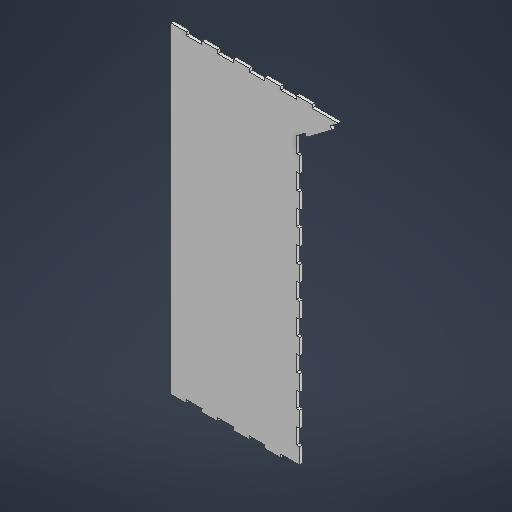
# Autodesk Inventor part: side
Saved by Autodesk Inventor 2026 (Build 300175050, 175E)
## iProperties
Created: 2025-08-08
Part Number: side
Material: Genérico
Document SubType Name: Modeling
Designer: EspacoMaker
Density: 1 g/cm^3
Appearance: Padrão
Author: EspacoMaker
Autodesk Inventor part; units mm, degrees
ref_plane "YZ Plane" through (0, 0, 0) normal (1, 0, 0) x (0, 1, 0)
ref_plane "XZ Plane" through (0, 0, 0) normal (0, 1, 0) x (-1, 0, 0)
ref_plane "XY Plane" through (0, 0, 0) normal (0, 0, 1) x (1, 0, 0)
sketch "Esboço1" plane through (0, 0, 0) normal (0, 0, 1) x (1, 0, 0)
  line L0 (60, -135) -> (-60, -135)
  line L1 (-60, -135) -> (-60, 135)
  line L2 (-60, 135) -> (60, 135)
  line L3 (60, 135) -> (60, -135)
  line L4 (60, -135) -> (-60, 135) construction
  line L5 (-60, -135) -> (60, 135) construction
  line L6 (-60, 135) -> (60, 135)
  line L7 (60, 135) -> (60, 165)
  line L8 (60, 165) -> (-60, 165)
  line L9 (-60, 165) -> (-60, 135)
  line L10 (60, 165) -> (100, 165)
  line L11 (100, 165) -> (60, 135)
  point P0 (0, 0)
  dimension "d0" = 120
  dimension "d1" = 270
  dimension "d2" = 120
  dimension "d3" = 30
  dimension "d4" = 40
  constraints: 24 end point, 4 parallel, 3 horizontal, 2 midpoint, 2 perpendicular
  measures "d0" distance of L1.end L2.end
  measures "d1" distance of L0.end L1.end
  measures "d2" distance of L8.end L7.end
  measures "d3" distance of L7.end L6.end
  measures "d4" distance of L7.end L10.end
extrude "Extrusão1" add sketch "Esboço1" along normal blind 3
sketch "Esboço2" plane through (60, -135, 0) normal (1, 0, 0) x (0, 0, -1)
  line L0 (-3, 0) -> (0, 0)
  line L1 (0, 0) -> (0, 15)
  line L2 (0, 15) -> (-3, 15)
  line L3 (-3, 15) -> (-3, 0)
  line L4 (-3, 30) -> (0, 30)
  line L5 (0, 30) -> (0, 45)
  line L6 (0, 45) -> (-3, 45)
  line L7 (-3, 45) -> (-3, 30)
  line L8 (-3, 60) -> (0, 60)
  line L9 (0, 60) -> (0, 75)
  line L10 (0, 75) -> (-3, 75)
  line L11 (-3, 75) -> (-3, 60)
  line L12 (-3, 90) -> (0, 90)
  line L13 (0, 90) -> (0, 105)
  line L14 (0, 105) -> (-3, 105)
  line L15 (-3, 105) -> (-3, 90)
  line L16 (-3, 120) -> (0, 120)
  line L17 (0, 120) -> (0, 135)
  line L18 (0, 135) -> (-3, 135)
  line L19 (-3, 135) -> (-3, 120)
  line L20 (-3, 150) -> (0, 150)
  line L21 (0, 150) -> (0, 165)
  line L22 (0, 165) -> (-3, 165)
  line L23 (-3, 165) -> (-3, 150)
  line L24 (-3, 180) -> (0, 180)
  line L25 (0, 180) -> (0, 195)
  line L26 (0, 195) -> (-3, 195)
  line L27 (-3, 195) -> (-3, 180)
  line L28 (-3, 210) -> (0, 210)
  line L29 (0, 210) -> (0, 225)
  line L30 (0, 225) -> (-3, 225)
  line L31 (-3, 225) -> (-3, 210)
  line L32 (-3, 240) -> (0, 240)
  line L33 (0, 240) -> (0, 255)
  line L34 (0, 255) -> (-3, 255)
  line L35 (-3, 255) -> (-3, 240)
  dimension "d7" = 3
  dimension "d8" = 15
  dimension "d11" = 30
  constraints: 72 end point, 2 parallel, 1 collinear, 1 horizontal, 1 perpendicular, 1 vertical, 63 other
  measures "d7" distance of L2.end L1.end
  measures "d8" distance of L1.end L0.end
  measures "d11" distance of L1.end L5.end
sketch "Esboço3" plane through (-60, -135, 0) normal (0, -1, 0) x (1, 0, 0)
  line L0 (160, 3) -> (0, 3) projected
  line L1 (0, 0) -> (15, 0)
  line L2 (15, 0) -> (15, 3)
  line L3 (15, 3) -> (0, 3)
  line L4 (0, 3) -> (0, 0)
  line L5 (30, 0) -> (45, 0)
  line L6 (45, 0) -> (45, 3)
  line L7 (45, 3) -> (30, 3)
  line L8 (60, 0) -> (75, 0)
  line L9 (75, 0) -> (75, 3)
  line L10 (75, 3) -> (60, 3)
  line L11 (90, 0) -> (105, 0)
  line L12 (105, 0) -> (105, 3)
  line L13 (105, 3) -> (90, 3)
  line L14 (30, 0) -> (45, 0)
  line L15 (45, 3) -> (30, 3)
  line L16 (45, 0) -> (45, 3)
  line L17 (30, 3) -> (30, 0)
  line L18 (60, 0) -> (75, 0)
  line L19 (75, 3) -> (60, 3)
  line L20 (75, 0) -> (75, 3)
  line L21 (60, 3) -> (60, 0)
  line L22 (90, 0) -> (105, 0)
  line L23 (105, 3) -> (90, 3)
  line L24 (105, 0) -> (105, 3)
  line L25 (90, 3) -> (90, 0)
  dimension "d16" = 15
  dimension "d17" = 3
  dimension "d20" = 30
  dimension "d27" = 30
  constraints: 50 end point, 3 horizontal, 2 parallel, 1 collinear, 1 perpendicular, 1 point on line, 44 other
  measures "d16" distance of L1.start L1.end
  measures "d17" distance of L1.end L2.end
  measures "d20" distance of L2.end L6.end
  measures "d27" distance of L1.start L14.start
sketch "Esboço4" plane through (-60, 165, 0) normal (0, 1, 0) x (1, 0, 0)
  line L0 (160, -3) -> (0, -3) projected
  line L1 (0, -3) -> (15, -3)
  line L2 (15, -3) -> (15, 0)
  line L3 (15, 0) -> (0, 0)
  line L4 (0, 0) -> (0, -3)
  line L5 (30, -3) -> (45, -3)
  line L6 (45, -3) -> (45, 0)
  line L7 (45, 0) -> (30, 0)
  line L8 (30, 0) -> (30, -3)
  line L9 (60, -3) -> (75, -3)
  line L10 (75, -3) -> (75, 0)
  line L11 (75, 0) -> (60, 0)
  line L12 (60, 0) -> (60, -3)
  line L13 (90, -3) -> (105, -3)
  line L14 (105, -3) -> (105, 0)
  line L15 (105, 0) -> (90, 0)
  line L16 (90, 0) -> (90, -3)
  line L17 (120, -3) -> (135, -3)
  line L18 (135, -3) -> (135, 0)
  line L19 (135, 0) -> (120, 0)
  line L20 (120, 0) -> (120, -3)
  point P0 (15, -3)
  dimension "d32" = 15
  dimension "d33" = 3
  dimension "d43" = 30
  constraints: 40 end point, 2 horizontal, 2 parallel, 1 perpendicular, 32 other
  measures "d32" distance of L2.end L3.end
  measures "d33" distance of L1.end L2.end
  measures "d43" distance of L2.end L6.end
sketch "Esboço5" plane through (100, 165, 0) normal (0.6, -0.8, 0) x (0.8, 0.6, 0)
  line L0 (0, 0) -> (-128, 0) projected
  line L1 (0, 0) -> (-10, 0)
  line L2 (-50, 0) -> (0, 0) projected
  line L3 (-10, 0) -> (-40, 0)
  line L4 (-40, 0) -> (-40, 3)
  line L5 (-40, 3) -> (-10, 3)
  line L6 (-10, 3) -> (-10, 0)
  point P0 (-179, 0)
  point P1 (-40, 0)
  dimension "d34" = 10
  dimension "d35" = 30
  dimension "d36" = 3
  constraints: 10 end point, 2 parallel, 1 horizontal, 1 perpendicular, 1 point on line
  measures "d34" distance of L0.start L1.end
  measures "d35" distance of L4.end L5.end
  measures "d36" distance of L3.end L4.end
extrude "Extrusão2" add sketch "Esboço2" along normal blind 3
extrude "Extrusão3" add sketch "Esboço3" along normal blind 3
extrude "Extrusão4" add sketch "Esboço4" along normal blind 3
extrude "Extrusão5" add sketch "Esboço5" along normal blind 3
equation "\"d16\" = d8"
equation "\"d17\" = d7"
equation "\"d32\" = d16"
equation "\"d33\" = d17"
equation "\"d36\" = d33"
